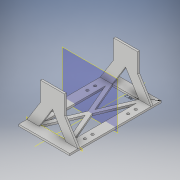
# Autodesk Inventor part: Square Support
Saved by Autodesk Inventor 2019 (Build 230136000, 136)
## iProperties
Created: 2019-04-16
Part Number: Square Support
Material: Generic
Document SubType Name: Modeling
Designer: kyle.fuchs
Density: 1 g/cm^3
Appearance: Default
Author: kyle.fuchs
Autodesk Inventor part; units mm, degrees
ref_plane "YZ Plane" through (0, 0, 0) normal (1, 0, 0) x (0, 1, 0)
ref_plane "XZ Plane" through (0, 0, 0) normal (0, 1, 0) x (-1, 0, 0)
sketch "Sketch1" plane through (0, 0, 0) normal (0, 1, 0) x (-1, 0, 0)
  line L0 (-127, 228.6) -> (-127, -228.6)
  line L1 (-65.8371, -177.8) -> (65.8371, -177.8)
  line L2 (127, -228.6) -> (127, 228.6)
  line L3 (65.8371, 177.8) -> (-65.8371, 177.8)
  line L4 (127, -228.6) -> (-127, -228.6)
  line L5 (-127, 228.6) -> (127, 228.6)
  line L6 (-76.2, 153.6199) -> (-76.2, -153.6199)
  line L7 (76.2, -153.6199) -> (76.2, 153.6199)
  line L8 (76.2, -153.6199) -> (10.3629, 0)
  line L9 (0, 24.1801) -> (-65.8371, 177.8)
  line L10 (65.8371, -177.8) -> (0, -24.1801)
  line L11 (-10.3629, 0) -> (-76.2, 153.6199)
  line L12 (76.2, 153.6199) -> (10.3629, 0)
  line L13 (0, -24.1801) -> (-65.8371, -177.8)
  line L14 (65.8371, 177.8) -> (0, 24.1801)
  line L15 (-10.3629, 0) -> (-76.2, -153.6199)
  point P0 (0, 0)
  point P1 (-127, 155.9501)
  point P2 (127, -155.9501)
  point P3 (-127, -155.9501)
  point P4 (127, 155.9501)
  constraints: 32 end point, 4 point on line, 2 parallel, 2 perpendicular, 1 vertical
extrude "Extrusion3" add sketch "Sketch1" along normal blind 9.525
sketch "Sketch7" plane through (0, 9.525, 0) normal (0, 1, 0) x (1, 0, 0)
  line L0 (0, 24.1801) -> (-65.8371, 177.8) projected
  line L1 (-127, 228.6) -> (-127, -228.6) projected
  line L2 (-76.2, 153.6199) -> (-76.2, -153.6199) projected
  circle A0 centre (-101.6, 127) radius 6.35
  circle A1 centre (-101.6, 88.9) radius 6.35
  line L3 (127, 228.6) -> (-127, 228.6) projected
  line L4 (-127, -228.6) -> (127, -228.6) projected
  circle A2 centre (101.6, 127) radius 6.35
  circle A3 centre (101.6, 88.9) radius 6.35
  line L5 (127, -228.6) -> (127, 228.6) projected
  circle A4 centre (-101.6, -127) radius 6.35
  circle A5 centre (-101.6, -88.9) radius 6.35
  circle A6 centre (101.6, -127) radius 6.35
  circle A7 centre (101.6, -88.9) radius 6.35
  point P0 (0, 0)
  constraints: 8 centre point
extrude "Extrusion4" cut sketch "Sketch7" against normal up to next contours A0 | A1 | A2 | A3 | A4 | A5 | A6 | A7
sketch "Sketch8" plane through (127, 0, -228.6) normal (0, 0, -1) x (-1, 0, 0)
  point P0 (127, 0)
ref_plane "Work Plane2" through (0, 0, 177.8) normal (0, 0, 1) x (1, 0, 0)
sketch "Sketch10" plane through (0, 0, 177.8) normal (0, 0, 1) x (1, 0, 0)
  line L0 (-127, 9.525) -> (127, 9.525) projected
  line L1 (0, 212.725) -> (-127, 9.525)
  line L2 (127, 0) -> (127, 9.525) projected
  line L3 (0, 212.725) -> (127, 9.525)
  line L4 (67.0942, 9.525) -> (0, 116.8758)
  line L5 (0, 116.8758) -> (-67.0942, 9.525)
  line L6 (-67.0942, 9.525) -> (-127, 9.525)
  line L7 (67.0942, 9.525) -> (127, 9.525)
  point P0 (0, 0)
  dimension "d35" = 50.8
  constraints: 12 end point, 3 point on line, 1 collinear
  measures "d35" distance between parallel lines of L1 L5
extrude "Extrusion5" add sketch "Sketch10" along normal blind 9.525 contours L1 L3 L0 L4 L5
mirror "Mirror2" about plane through (0, 0, 0) normal (0, 0, 1) of "Extrusion5"
sketch "Sketch11" plane through (-67.0942, 9.525, -187.325) normal (0, 0, -1) x (-1, 0, 0)
  line L0 (-67.0942, 107.3508) -> (-134.1884, 0) projected
  line L1 (-67.0942, 203.2) -> (59.9058, 0) projected
  line L2 (0, 0) -> (-67.0942, 107.3508) projected
  line L3 (-67.0942, 107.3508) -> (-7.1884, 107.3508)
  line L4 (-67.0942, 203.2) -> (59.9058, 0) projected
  line L5 (-7.1884, 203.2) -> (-67.0942, 203.2)
  line L6 (-7.1884, 203.2) -> (-7.1884, 107.3508)
  line L7 (-67.0942, 107.3508) -> (-127, 107.3508)
  line L8 (-194.0942, 0) -> (-67.0942, 203.2) projected
  line L9 (-127, 107.3508) -> (-127, 203.2)
  line L10 (-127, 203.2) -> (-67.0942, 203.2)
  line L11 (-7.1884, 155.2754) -> (-127, 155.2754)
  point P0 (-67.0942, -9.525)
  constraints: 14 end point, 4 point on line, 2 horizontal, 2 midpoint, 1 parallel, 1 perpendicular, 1 vertical
extrude "Extrusion6" add sketch "Sketch11" against normal blind 9.525 contours L5 L6 L11 L1 | L8 L11 L9 L10 | L11 L6 L1 | L8 L9 L11
mirror "Mirror3" about plane through (0, 0, 0) normal (0, 0, 1) of "Extrusion6", "Extrusion5", "Mirror2"
ref_plane "Work Plane3" through (0, 0, 0) normal (0, 0, 1) x (1, 0, 0)
body "Solid2"
